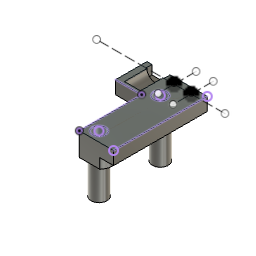
power_tray v7 (Autodesk Fusion 360 design; units mm, degrees)
Autodesk Fusion 360 part; units mm, degrees
sketch "Skizze1" plane through (0, 0, 0) normal (0, 0, 1) x (1, 0, 0)
  line L0 (12, -20) -> (-18, -20)
  line L1 (-18, -20) -> (-18, 26.6)
  line L2 (-18, 26.6) -> (12, 26.6)
  line L3 (12, 26.6) -> (12, -20)
  line L4 (-36.0472, 15.24) -> (32.5304, 15.24) construction
  line L5 (-35.3146, -15.24) -> (27.6948, -15.24) construction
  circle A0 centre (0, 15.24) radius 4
  circle A1 centre (0, -15.24) radius 4
  line L6 (-5, -20) -> (-5, 11)
  line L7 (-5, 11) -> (-18, 11)
  circle A2 centre (0, 15.24) radius 7
  circle A3 centre (0, -15.24) radius 7
  line L8 (0, 19) -> (0, -24.3873) construction
  point P0 (0, 15.24)
  point P1 (0, -15.24)
  dimension "d3" = 20
  dimension "d4" = 26.6
  dimension "d5" = 12
  dimension "d6" = 18
  dimension "d7" = 15.24
  dimension "d8" = 15.24
  dimension "d9" = 8
  dimension "d10" = 8
  dimension "d45" = 13
  dimension "d46" = 31
  dimension "d47" = 14
  dimension "d48" = 14
  constraint horizontal L0
  constraint vertical L1
  constraint horizontal L2
  constraint vertical L3
  constraint horizontal L4
  constraint horizontal L5
  constraint coincident L4 P0
  constraint coincident L5 P1
  constraint coincident P0 A0.centre
  constraint coincident P1 A1.centre
  constraint coincident L0 L6.start
  constraint perpendicular L0 L6
  constraint coincident L1 L7.end
  constraint perpendicular L1 L7
  constraint concentric A0 A2
  constraint concentric A1 A3
  constraint vertical L8
  constraint coincident origin L8
  constraint coincident P0 L8
  constraint coincident P1 L8
  measures "d3" distance of origin L0
  measures "d4" distance of origin L2
  measures "d5" distance of origin L3
  measures "d6" distance of origin L1
  measures "d7" distance of origin L4
  measures "d8" distance of origin L5
  measures "d9" diameter of A0
  measures "d10" diameter of A1
  measures "d45" distance of L1 L6
  measures "d46" distance of L0 L7
  measures "d47" diameter of A3
  measures "d48" diameter of A2
extrude "Extrusion1" add sketch "Skizze1" along normal blind 6.5 contours L0 L1 L2 L3 L6 L7 A2 A3 | L0 L6 A3 | L6 L7 A2 | A0 | A1 picked at (-4.6667, -15.1937) picked at (-3.9058, 10.9235)
sketch "Skizze2" plane through (0, 26.6, 0) normal (0, 1, 0) x (-1, 0, 0)
  line L0 (-12, 0) -> (18, 0)
  line L1 (18, 0) -> (18, 6.5)
  line L2 (18, 6.5) -> (-12, 6.5)
  line L3 (-12, 6.5) -> (-12, 0)
  line L4 (11, 13.5) -> (11, -12.5) construction
  line L5 (6.5, 6.5) -> (15.5, 6.5)
  line L6 (15.5, 6.5) -> (15.5, 2)
  line L7 (15.5, 2) -> (6.5, 2)
  line L8 (6.5, 2) -> (6.5, 6.5)
  line L9 (7, 8.5) -> (7, -2.5) construction
  line L10 (15, 8.4924) -> (15, -3.3602) construction
  arc A0 (7, 6.5) -> (15, 6.5) centre (11, 6.5) ccw
  point P0 (7, 6.5)
  point P1 (7, 6.5)
  point P2 (11, 6.5)
  dimension "d13" = 7
  dimension "d14" = 4.5
  dimension "d15" = 4.5
  dimension "d16" = 4.5
  dimension "d17" = 4
  dimension "d18" = 4
  constraint vertical L4
  constraint horizontal L5
  constraint vertical L6
  constraint horizontal L7
  constraint vertical L8
  constraint coincident L2 L5.start
  constraint perpendicular L0 L9
  constraint perpendicular L5 L10
  constraint coincident L5 P1
  constraint coincident L9 P1
  constraint coincident L2 P1
  constraint midpoint L5 P2
  constraint coincident P1 P0
  constraint coincident P2 A0.centre
  measures "d13" distance of L1 L4
  measures "d14" distance of L4 L8
  measures "d15" distance of L4 L6
  measures "d16" distance of L5 L7
  measures "d17" distance of L4 L9
  measures "d18" distance of L4 L10
extrude "Extrusion2" cut sketch "Skizze2" against normal blind 3 contours L2 L5 L6 L7 L8 A0
extrude "Extrusion3" cut sketch "Skizze2" against normal blind 14.2 contours L2 L5 A0
extrude "Extrusion6" add sketch "Skizze1" against normal blind 5 contours L0 L6 A3 picked at (-4.6667, -15.1937)
extrude "Extrusion7" add sketch "Skizze1" against normal blind 5 contours L6 L7 A2 picked at (-3.9058, 10.9235)
extrude "Extrusion4" add sketch "Skizze1" against normal blind 21.5 contours A0 | A1
sketch "Skizze3" plane through (0, 0, -21.5) normal (0, 0, -1) x (1, 0, 0)
  circle A0 centre (0, -15.24) radius 4
  line L0 (0, -27) -> (0, 23.61) construction
  line L1 (21.7334, -15.24) -> (-22.4317, -15.24) construction
  line L2 (22.3444, 15.24) -> (-24, 15.24) construction
  point P0 (0, -15.24)
  point P1 (0, 15.24)
  dimension "d25" = 15.24
  dimension "d26" = 15.24
  constraint vertical L0
  constraint horizontal L1
  constraint horizontal L2
  constraint coincident P0 A0.centre
  constraint coincident L2 P1
  constraint coincident L0 P1
  measures "d25" distance of L1 origin
  measures "d26" distance of L2 origin
hole "Bohrung1" at (0, 15.24, -21.5) at (0, -15.24, -21.5) direction (0, 0, 1) diameter 3.5 depth 30 tip angle 180
sketch "Skizze6" plane through (0, 0, 6.5) normal (0, 0, 1) x (-1, 0, 0)
  line L0 (15, -12.4) -> (15, -23.6)
  line L1 (15, -23.6) -> (15.5, -23.6)
  line L2 (15.5, -23.6) -> (15.5, -26.6)
  line L3 (15.5, -26.6) -> (18, -26.6)
  line L4 (18, -26.6) -> (18, -11)
  line L5 (18, -11) -> (5, -11)
  line L6 (5, -11) -> (5, 20)
  line L7 (5, 20) -> (-12, 20)
  line L8 (-12, 20) -> (-12, -26.6)
  line L9 (-12, -26.6) -> (6.5, -26.6)
  line L10 (6.5, -26.6) -> (6.5, -23.6)
  line L11 (6.5, -23.6) -> (7, -23.6)
  line L12 (7, -23.6) -> (7, -12.4)
  line L13 (7, -12.4) -> (15, -12.4)
  line L14 (22.7431, -15.24) -> (-23, -15.24) construction
  line L15 (16, 15.24) -> (-23, 15.24) construction
  line L16 (0, -29.9031) -> (0, 26.376) construction
  circle A0 centre (0, -15.24) radius 1.75
  circle A1 centre (0, 15.24) radius 1.75
  point P0 (0, -15.24)
  point P1 (0, 15.24)
  dimension "d53" = 15.24
  dimension "d54" = 15.24
  constraint horizontal L14
  constraint perpendicular L6 L15
  constraint vertical L16
  constraint coincident origin L16
  constraint coincident L14 P0
  constraint coincident L16 P0
  measures "d53" distance of origin L14
  measures "d54" distance of origin L15
hole "Bohrung3" at (0, 15.24, 6.5) at (0, -15.24, 6.5) direction (0, 0, -1) diameter 6.5 depth 6.5 tip angle 90
sketch "Skizze4" plane through (0, 0, 6.5) normal (0, 0, 1) x (-1, 0, 0)
  line L0 (15, -12.4) -> (15, -23.6)
  line L1 (15, -23.6) -> (15.5, -23.6)
  line L2 (15.5, -23.6) -> (15.5, -26.6)
  line L3 (15.5, -26.6) -> (18, -26.6)
  line L4 (18, -26.6) -> (18, -11)
  line L5 (5, 20) -> (-12, 20)
  line L6 (-12, 20) -> (-12, -26.6)
  line L7 (-12, -26.6) -> (6.5, -26.6)
  line L8 (6.5, -26.6) -> (6.5, -23.6)
  line L9 (6.5, -23.6) -> (7, -23.6)
  line L10 (7, -23.6) -> (7, -12.4)
  line L11 (7, -12.4) -> (15, -12.4)
  line L12 (-23.7996, -23.6) -> (40, -23.6) construction
  line L13 (-7, -34.5714) -> (-7, -14.6073) construction
  line L14 (1.5, -34.5334) -> (1.5, -15.6973) construction
  line L15 (-12, -26.6) -> (-12, 20)
  line L16 (18, -11) -> (5, -11)
  line L17 (5, -11) -> (5, 20)
  circle A0 centre (0, -15.24) radius 3.25
  circle A1 centre (0, 15.24) radius 3.25
  point P0 (-7, -23.6)
  point P1 (1.5, -23.6)
  dimension "d30" = 3
  dimension "d31" = 5
  dimension "d32" = 5
  dimension "d33" = 8.5
  constraint horizontal L12
  constraint perpendicular L7 L13
  constraint parallel L6 L14
  constraint coincident L12 P0
  constraint coincident L13 P0
  constraint coincident L14 P1
  constraint coincident L12 P1
  measures "d30" distance of L6.end L12
  measures "d31" distance of L13 L15
  measures "d32" distance of L8 L14
  measures "d33" distance of L13 L14
hole "Bohrung2" at (7, 23.6, 6.5) at (-1.5, 23.6, 6.5) direction (0, 0, -1) diameter 2.5 depth 8 tip angle 180
ref_plane "Arbeitsebene1" through (0, 0, 2.7) normal (0, 0, 1) x (1, 0, 0)
sketch "Skizze5" plane through (0, 0, 2.7) normal (0, 0, 1) x (1, 0, 0)
  line L0 (18, 23.6) -> (-21, 23.6) construction
  line L1 (-18, 26.6) -> (12, 26.6)
  line L2 (7, 19.6167) -> (7, 31.5736) construction
  line L3 (-1.5, 19.6924) -> (-1.5, 31.9243) construction
  line L4 (12, 26.6) -> (12, -20)
  line L5 (5.7298, 25.8) -> (4.4597, 23.6)
  line L6 (4.4597, 23.6) -> (5.7298, 21.4)
  line L7 (5.7298, 21.4) -> (8.2702, 21.4)
  line L8 (8.2702, 21.4) -> (9.5403, 23.6)
  line L9 (9.5403, 23.6) -> (8.2702, 25.8)
  line L10 (8.2702, 25.8) -> (5.7298, 25.8)
  line L11 (-2.7702, 25.8) -> (-4.0403, 23.6)
  line L12 (-4.0403, 23.6) -> (-2.7702, 21.4)
  line L13 (-2.7702, 21.4) -> (-0.2298, 21.4)
  line L14 (-0.2298, 21.4) -> (1.0403, 23.6)
  line L15 (1.0403, 23.6) -> (-0.2298, 25.8)
  line L16 (-0.2298, 25.8) -> (-2.7702, 25.8)
  point P0 (7, 23.6)
  point P1 (-1.5, 23.6)
  dimension "d38" = 3
  dimension "d39" = 5
  dimension "d40" = 8.5
  dimension "d41" = 4.4
  dimension "d42" = 4.4
  constraint horizontal L0
  constraint vertical L2
  constraint vertical L3
  constraint coincident L0 P0
  constraint coincident L2 P0
  constraint midpoint L0 P1
  measures "d38" distance of L0 L1
  measures "d39" distance of L2 L4
  measures "d40" distance of L2.end L3
  measures "d41" distance of L7 L10
  measures "d42" distance of L13 L16
extrude "Extrusion5" cut sketch "Skizze5" along normal blind 1.8
